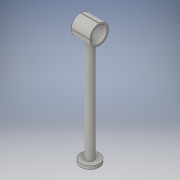
# Autodesk Inventor part: piston2
Saved by Autodesk Inventor 2016 (Build 200138000, 138)
## iProperties
Created: 2018-01-12
Part Number: piston2
Material: Generic
Document SubType Name: Modeling
Designer: New User
Density: 1 g/cm^3
Appearance: Default
Author: New User
Autodesk Inventor part; units mm, degrees
ref_plane "YZ Plane" through (0, 0, 0) normal (1, 0, 0) x (0, 1, 0)
ref_plane "XZ Plane" through (0, 0, 0) normal (0, 1, 0) x (-1, 0, 0)
ref_plane "XY Plane" through (0, 0, 0) normal (0, 0, 1) x (1, 0, 0)
sketch "Sketch1" plane through (0, 0, 0) normal (0, 1, 0) x (-1, 0, 0)
  circle A0 centre (0, 0) radius 3.683
  dimension "d0" = 7.366
  constraints: 1 centre point, 1 coincident
  measures "d0" diameter of A0
extrude "Extrusion1" add sketch "Sketch1" along normal blind 1.27
sketch "Sketch2" plane through (0, 1.27, 0) normal (0, 1, 0) x (1, 0, 0)
  circle A0 centre (0, 0) radius 1.5875
  dimension "d3" = 3.175
  constraints: 1 centre point, 1 coincident
  measures "d3" diameter of A0
extrude "Extrusion2" add sketch "Sketch2" along normal blind 40.64
sketch "Sketch3" plane through (0, 41.91, 0) normal (0, 1, 0) x (1, 0, 0)
  line L0 (3.683, 3.683) -> (-3.683, 3.683)
  line L1 (-3.683, 3.683) -> (-3.683, -3.683)
  line L2 (-3.683, -3.683) -> (3.683, -3.683)
  line L3 (3.683, -3.683) -> (3.683, 3.683)
  line L4 (3.683, 3.683) -> (-3.683, -3.683) construction
  line L5 (-3.683, 3.683) -> (3.683, -3.683) construction
  point P0 (0, 0)
  constraints: 12 end point, 2 midpoint, 2 parallel, 1 horizontal, 1 perpendicular
extrude "Extrusion3" add sketch "Sketch3" along normal blind 7.62
sketch "Sketch4" plane through (3.683, 41.91, 3.683) normal (1, 0, 0) x (0, 0, -1)
  circle A0 centre (3.556, 3.81) radius 3.175
  line L0 (7.366, 7.62) -> (0, 7.62) projected
  line L1 (7.366, 0) -> (7.366, 7.62) projected
  point P0 (3.683, -41.91)
  dimension "d8" = 3.81
  dimension "d9" = 3.81
  dimension "d10" = 6.35
  constraints: 1 centre point
  measures "d8" distance from line of L0 A0.centre
  measures "d9" distance from line of L1 A0.centre
  measures "d10" diameter of A0
extrude "Extrusion4" cut sketch "Sketch4" against normal blind 7.62
fillet "Fillet1" radius 3.556 4 edges at (0, 41.91, 3.683) (0, 49.53, 3.683) (0, 49.53, -3.683) (0, 41.91, -3.683)
body "Solid1"
